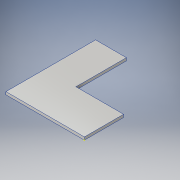
# Autodesk Inventor part: RSX bottom
Saved by Autodesk Inventor 2016 (Build 200138000, 138)
## iProperties
Created: 2017-04-05
Part Number: RSX bottom
Material: Aluminum 6061
Document SubType Name: Modeling
Designer: Ethan
Density: 2.7 g/cm^3
Appearance: Aluminum - Flat
Mass: 407.884 g
Surface Area: 524.192 cm^2
Volume: 151.068 cm^3
Author: Ethan
Autodesk Inventor part; units mm, degrees
ref_plane "YZ Plane" through (0, 0, 0) normal (1, 0, 0) x (0, 1, 0)
ref_plane "XZ Plane" through (0, 0, 0) normal (0, 1, 0) x (-1, 0, 0)
ref_plane "XY Plane" through (0, 0, 0) normal (0, 0, 1) x (1, 0, 0)
sketch "Sketch1" plane through (0, 0, 0) normal (0, 1, 0) x (-1, 0, 0)
  point P0 (0, 0)
sketch "Sketch2" plane through (0, 0, 0) normal (0, 1, 0) x (-1, 0, 0)
  line L0 (0, 0) -> (177.8, 0)
  line L1 (177.8, 0) -> (177.8, -203.2)
  line L2 (0, 0) -> (0, -88.9)
  line L3 (177.8, -203.2) -> (107.95, -203.2)
  line L4 (107.95, -203.2) -> (107.95, -88.9)
  line L5 (0, -88.9) -> (107.95, -88.9)
  dimension "d0" = 203.2
  dimension "d1" = 177.8
  dimension "d2" = 88.9
  dimension "d3" = 69.85
  constraints: 12 end point, 3 horizontal, 1 perpendicular, 1 vertical
  measures "d0" distance of L0.end L1.end
  measures "d1" distance of L0.start L0.end
  measures "d2" distance of L0.start L2.end
  measures "d3" distance of L1.end L3.end
extrude "Extrusion1" add sketch "Sketch2" along normal blind 6.35
body "Solid1"
